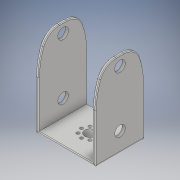
# Autodesk Inventor part: Wheel Case V3
Saved by Autodesk Inventor 2019 (Build 230136000, 136)
## iProperties
Created: 2018-12-01
Part Number: Wheel Case V3
Material: Generic
Document SubType Name: Modeling
Designer: Ashley
Density: 1 g/cm^3
Appearance: Default
Author: Ashley
Autodesk Inventor part; units mm, degrees
ref_plane "YZ Plane" through (0, 0, 0) normal (1, 0, 0) x (0, 1, 0)
ref_plane "XZ Plane" through (0, 0, 0) normal (0, 1, 0) x (-1, 0, 0)
ref_plane "XY Plane" through (0, 0, 0) normal (0, 0, 1) x (1, 0, 0)
sketch "Sketch1" plane through (0, 0, 0) normal (0, 1, 0) x (-1, 0, 0)
  line L0 (40, 32.5) -> (-40, 32.5)
  line L1 (-40, 32.5) -> (-40, -32.5)
  line L2 (-40, -32.5) -> (40, -32.5)
  line L3 (40, -32.5) -> (40, 32.5)
  line L4 (40, 32.5) -> (-40, -32.5) construction
  line L5 (-40, 32.5) -> (40, -32.5) construction
  point P0 (0, 0)
  dimension "d0" = 80
  dimension "d1" = 65
  constraints: 12 end point, 2 midpoint, 2 parallel, 1 horizontal, 1 perpendicular
  measures "d0" distance of L1.end L2.end
  measures "d1" distance of L0.end L1.end
extrude "Top Base Extrusion" add sketch "Sketch1" along normal blind 4
sketch "Sketch2" plane through (0, 4, 0) normal (0, 1, 0) x (1, 0, 0)
  line L0 (-40, -32.5) -> (40, -32.5) construction
  line L1 (40, -32.5) -> (40, 32.5) construction
  line L2 (-40, 32.5) -> (-40, -32.5) construction
  line L3 (-40, 32.5) -> (-36, 32.5)
  line L4 (-36, 32.5) -> (-36, -32.5)
  line L5 (-36, -32.5) -> (-40, -32.5)
  line L6 (-40, -32.5) -> (-40, 32.5)
  line L7 (40, 32.5) -> (36, 32.5)
  line L8 (36, 32.5) -> (36, -32.5)
  line L9 (36, -32.5) -> (40, -32.5)
  line L10 (40, -32.5) -> (40, 32.5)
  point P0 (0, 0)
  dimension "d4" = 4
  dimension "d5" = 4
  constraints: 16 end point, 4 parallel, 2 horizontal, 2 perpendicular, 2 point on line
  measures "d4" distance between parallel lines of L4 L2
  measures "d5" distance between parallel lines of L1 L8
extrude "Side Extrusions" add sketch "Sketch2" along normal blind 110
sketch "Sketch3" plane through (40, 0, 32.5) normal (1, 0, 0) x (0, 0, -1)
  circle A0 centre (32.5, 101.5) radius 7.1
  circle A1 centre (32.5, 26.5) radius 7
  line L0 (65, 0) -> (65, 114) construction
  line L1 (0, 114) -> (65, 114) construction
  line L2 (0, 0) -> (0, 114) construction
  line L3 (0, 4) -> (65, 4) construction
  point P0 (32.5, 0)
  dimension "d8" = 14.2
  dimension "d11" = 101.5
  dimension "d43" = 75
  dimension "d44" = 14
  dimension "d45" = 65
  dimension "d46" = 32.5
  dimension "d47" = 32.5
  dimension "d48" = 32.5
  dimension "d49" = 12.5
  dimension "d50" = 22.5
  constraints: 2 centre point
  measures "d8" diameter of A0
  measures "d11" distance of point (32.5, 0) A0.centre
  measures "d43" distance of A1.centre A0.centre
  measures "d44" diameter of A1
  measures "d45" distance between parallel lines of L2 L0
  measures "d46" distance from line of L0 A0.centre
  measures "d47" distance from line of L2 A0.centre
  measures "d48" distance from line of L0 A1.centre
  measures "d49" distance from line of A0.centre L1
  measures "d50" distance from line of A1.centre L3
extrude "Wheel Axel Hole" cut sketch "Sketch3" against normal up to surface (80 mm away)
sketch "Sketch4" plane through (0, 0, 0) normal (0, -1, 0) x (1, 0, 0)
  circle A0 centre (0, 0) radius 7.1
  circle A1 centre (0, 0) radius 16
  dimension "d16" = 14.2
  dimension "d17" = 32
  constraints: 2 centre point, 2 coincident
  measures "d16" diameter of A0
  measures "d17" diameter of A1
extrude "Chain Interferance Extrusion" add sketch "Sketch4" along normal blind 6
sketch "Sketch5" plane through (0, 0, 0) normal (0, -1, 0) x (1, 0, 0)
  circle A0 centre (0, 0) radius 7.1 construction
  circle A1 centre (0, 0) radius 7.1
  constraints: 1 centre point, 1 coincident, 1 concentric
extrude "Top Center Bearing Hole" cut sketch "Sketch5" against normal up to surface (4 mm away)
sketch "Sketch7" plane through (0, -6, 0) normal (0, -1, 0) x (1, 0, 0)
  circle A0 centre (0, 0) radius 7.1 construction
  circle A1 centre (0, 11.314) radius 2.05
  circle A2 centre (-8.0002, 8.0002) radius 2.05
  circle A3 centre (-11.314, 0) radius 2.05
  circle A4 centre (-8.0002, -8.0002) radius 2.05
  circle A5 centre (0, -11.314) radius 2.05
  circle A6 centre (8.0002, -8.0002) radius 2.05
  circle A7 centre (11.314, 0) radius 2.05
  circle A8 centre (8.0002, 8.0002) radius 2.05
  dimension "d23" = 4.1
  dimension "d24" = 11.314
  dimension "d27" = 360
  constraints: 8 centre point, 17 other
  measures "d23" diameter of A1
  measures "d24" distance of A0.centre A1.centre
extrude "Sprocket Screws Holes" cut sketch "Sketch7" against normal up to next
sketch "Sketch8" plane through (40, 0, 32.5) normal (1, 0, 0) x (0, 0, -1)
  line L0 (65, 0) -> (65, 114) construction
  line L1 (0, 114) -> (65, 114) construction
  line L2 (0, 0) -> (0, 114) construction
  line L3 (65, 91.5) -> (52.0096, 114)
  line L4 (65, 114) -> (0, 114) construction
  line L5 (65, 91.5) -> (90.9808, 91.5) construction
  line L6 (0, 91.5) -> (34.6363, 91.5) construction
  line L7 (0, 91.5) -> (44.4453, 91.5) construction
  line L8 (0, 91.5) -> (12.9904, 114)
  line L9 (65, 91.5) -> (65, 114)
  line L10 (52.0096, 114) -> (65, 114)
  line L11 (12.9904, 114) -> (0, 114)
  line L12 (0, 91.5) -> (0, 114)
  line L13 (0, 91.5) -> (-31.251, 91.5) construction
  point P0 (32.5, 0)
  dimension "d32" = 120
  dimension "d51" = 120
  constraints: 20 end point, 5 point on line, 3 collinear, 3 horizontal, 1 equal length, 1 perpendicular
  measures "d32" angle of L5 L3
  measures "d51" angle of L13 L8
extrude "Side Corners Cut" cut sketch "Sketch8" against normal up to surface (80 mm away)
fillet "Fillet1" radius 95 4 edges at (38, 91.5, 32.5) (-38, 91.5, 32.5) (38, 91.5, -32.5) (-38, 91.5, -32.5)
fillet "Fillet2" radius 23 4 edges at (38, 114, 19.5096) (38, 114, -19.5096) (-38, 114, -19.5096) (-38, 114, 19.5096)
fillet "Fillet3" radius 3 4 edges at (0, 0, -32.5) (-40, 0, 0) (40, 0, 0) (0, 0, 32.5)
fillet "Fillet4" radius 3 1 edges at (-16, 0, 0)
fillet "Fillet5" radius 1 1 edges at (-16, -6, 0)
fillet "Fillet7" radius 1 34 edges at (40, 109.8726, 18.1832) (40, 114, 0) (40, 109.8726, -18.1832) (40, 82.7695, -31.0162) (40, 34.5224, -32.5) (39.1213, 0.8787, -31.6213) (40, 34.5224, 32.5) (39.1213, 0.8787, 31.6213) (40, 82.7695, 31.0162) (36, 35.0224, 32.5) (36, 109.8726, 18.1832) (36, 114, 0) (36, 109.8726, -18.1832) (36, 82.7695, -31.0162) (36, 35.0224, -32.5) (36, 82.7695, 31.0162) (-36, 109.8726, 18.1832) (-36, 114, 0) (-36, 109.8726, -18.1832) (-36, 82.7695, -31.0162) (-36, 35.0224, -32.5) (-36, 35.0224, 32.5) (-36, 82.7695, 31.0162) (-40, 34.5224, 32.5) (-39.1213, 0.8787, 31.6213) (-40, 109.8726, 18.1832) (-40, 114, 0) (-40, 109.8726, -18.1832) (-40, 82.7695, -31.0162) (-40, 34.5224, -32.5) (-39.1213, 0.8787, -31.6213) (-40, 82.7695, 31.0162) (0, 4, 32.5) (0, 4, -32.5)
body "Solid1"
